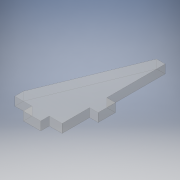
# Autodesk Inventor part: Belt_Holder3
Saved by Autodesk Inventor 2016 (Build 200138000, 138)
## iProperties
Created: 2018-06-03
Part Number: Belt_Holder3
Material: Polycarbonate, Clear
Document SubType Name: Modeling
Designer: Phil Erle
Density: 1.2 g/cm^3
Appearance: Polycarbonate - Clear
Author: Phil Erle
Autodesk Inventor part; units mm, degrees
ref_plane "YZ Plane" through (0, 0, 0) normal (1, 0, 0) x (0, 1, 0)
ref_plane "XZ Plane" through (0, 0, 0) normal (0, 1, 0) x (-1, 0, 0)
ref_plane "XY Plane" through (0, 0, 0) normal (0, 0, 1) x (1, 0, 0)
sketch "Sketch1" plane through (0, 0, 0) normal (0, 0, 1) x (1, 0, 0)
  line L0 (-27.5, 0) -> (-27.5, 5)
  line L1 (-27.5, 5) -> (-5, 60)
  line L2 (-5, 60) -> (0, 60)
  line L3 (-27.5, 0) -> (-17.5, 0)
  line L4 (-17.5, 0) -> (-17.5, -5)
  line L5 (-17.5, -5) -> (-7.5, -5)
  line L6 (-7.5, -5) -> (-7.5, 0)
  line L7 (-7.5, 0) -> (0, 0)
  line L8 (0, 60) -> (0, 26)
  line L9 (0, 26) -> (5, 26)
  line L10 (5, 26) -> (5, 16)
  line L11 (5, 16) -> (0, 16)
  line L12 (0, 16) -> (0, 0)
  dimension "d0" = 5
  dimension "d1" = 5
  dimension "d2" = 27.5
  dimension "d3" = 60
  dimension "d4" = 10
  dimension "d5" = 10
  dimension "d6" = 10
  dimension "d7" = 5
  dimension "d8" = 16
  dimension "d9" = 5
  dimension "d11" = 90
  constraints: 26 end point, 8 perpendicular, 2 point on line, 1 horizontal, 1 vertical
  measures "d0" distance of L1.end L2.end
  measures "d1" distance of L0.start L0.end
  measures "d2" distance of L7.end L0.start
  measures "d3" distance of L2.end L7.end
  measures "d4" distance of L4.end L5.end
  measures "d5" distance between parallel lines of L0 L4
  measures "d6" distance of L9.end L10.end
  measures "d7" distance of L8.end L9.end
  measures "d8" distance between parallel lines of L7 L11
  measures "d9" distance of L5.end L6.end
  measures "d11" angle of L8 L2
extrude "Extrusion1" add sketch "Sketch1" along normal blind 5
body "Solid1"
